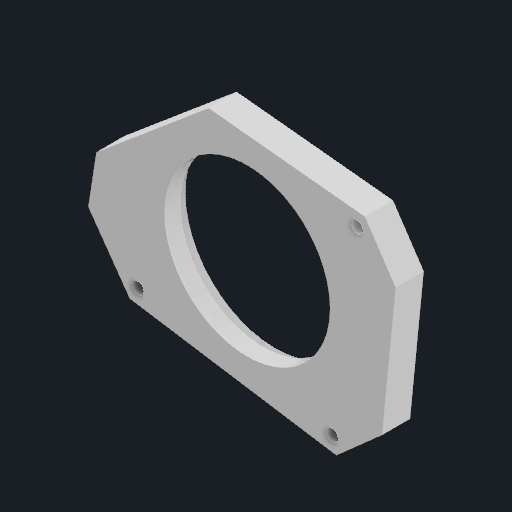
# Autodesk Inventor part: TongueSideLid
Saved by Autodesk Inventor 2025.2 (Build 292293000, 293)
## iProperties
Created: 2024-12-20
Part Number: TongueSideLid
Material: Generic
Document SubType Name: Modeling
Designer: valer
Density: 1 g/cm^3
Appearance: Default
Author: valer
Autodesk Inventor part; units mm, degrees
ref_plane "YZ Plane" through (0, 0, 0) normal (1, 0, 0) x (0, 1, 0)
ref_plane "XZ Plane" through (0, 0, 0) normal (0, 1, 0) x (-1, 0, 0)
ref_plane "XY Plane" through (0, 0, 0) normal (0, 0, 1) x (1, 0, 0)
sketch "Sketch1" plane through (0, 0, 0) normal (0, 0, 1) x (1, 0, 0)
  line L0 (0.6045, 32.7277) -> (-43.9747, 37.2532) construction
  line L1 (-49.7733, -7.6646) -> (-5.5064, -14.6087) construction
  circle A0 centre (-43.015, 34.1404) radius 3.175 construction
  line L2 (-5.5064, -14.6087) -> (15.1919, 3.7419) construction
  line L3 (-42.0553, 31.0275) -> (-2.8152, 27.0441) construction
  line L4 (-7.3705, -8.2429) -> (-46.3358, -2.1305) construction
  line L5 (9.5291, 6.74) -> (-7.3705, -8.2429) construction
  line L6 (-2.8152, 27.0441) -> (9.7254, 8.2606) construction
  line L7 (-32.8846, 36.1274) -> (0.6045, 32.7277)
  line L8 (-32.8846, 36.1274) -> (-56.9375, 15.8971)
  line L9 (-65.2029, 14.1906) -> (-49.7733, -7.6646) construction
  line L10 (15.9639, 9.7222) -> (0.6045, 32.7277) construction
  line L11 (0.6045, 32.7277) -> (7.1877, 22.8674)
  line L12 (7.1877, 22.8674) -> (4.2625, -5.9478)
  line L13 (4.2625, -5.9478) -> (-5.5064, -14.6087)
  line L14 (-5.5064, -14.6087) -> (-49.7733, -7.6646)
  line L15 (-49.7733, -7.6646) -> (-58.6592, 4.9218)
  line L16 (-56.9375, 15.8971) -> (-58.6592, 4.9218)
  line L17 (-58.7974, 16.9461) -> (-42.0553, 31.0275) construction
  circle A1 centre (-24.6239, 11.922) radius 17.75
  circle A2 centre (-1.1053, 29.8859) radius 1.25
  circle A3 centre (-48.0546, -4.8975) radius 1.25
  circle A4 centre (-6.4384, -11.4258) radius 1.25
  point P0 (0, 0)
  dimension "d0" = 2
  dimension "d1" = 2
  dimension "d2" = 4
  constraints: 36 end point, 7 collinear, 5 centre point, 2 perpendicular, 1 parallel, 1 point on line, 34 other
  measures "d0" distance between parallel lines of L17 L8
  measures "d1" distance from line of L16 L17.start
  measures "d2" distance from line of L6.end L12
extrude "Extrusion1" add sketch "Sketch1" along normal blind 6
sketch "Sketch2" plane through (0, 0, 0) normal (0, 0, -1) x (-1, 0, 0)
  circle A0 centre (24.6239, 11.922) radius 17.75 projected
  circle A1 centre (24.6239, 11.922) radius 19.25
  point P0 (0, 0)
  dimension "d5" = 38.5
  constraints: 1 centre point, 1 coincident
  measures "d5" diameter of A1
extrude "Extrusion2" cut sketch "Sketch2" against normal blind 2.5
equation "\"d1\" = d0"
body "Solid1"
